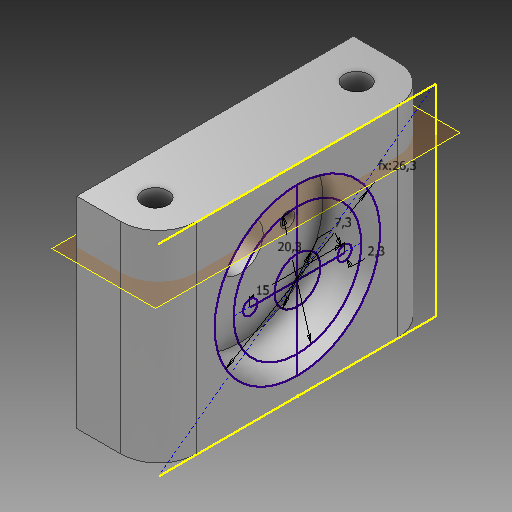
# Autodesk Inventor part: motor_mount_edge
Saved by Autodesk Inventor 2020 (Build 240168000, 168)
## iProperties
Created: 2024-09-09
Part Number: motor_mount_edge
Material: Типовые
Document SubType Name: Modeling
Designer: Ivan
Density: 1 g/cm^3
Appearance: Анодированный — светло-серый
Высота: 32,000 мм
Author: Ivan
Autodesk Inventor part; units mm, degrees
ref_plane "YZ Plane" through (0, 0, 0) normal (1, 0, 0) x (0, 1, 0)
ref_plane "XZ Plane" through (0, 0, 0) normal (0, 1, 0) x (-1, 0, 0)
ref_plane "XY Plane" through (0, 0, 0) normal (0, 0, 1) x (1, 0, 0)
sketch "Эскиз1" plane through (0, 0, 0) normal (0, 1, 0) x (-1, 0, 0)
  line L0 (6.5, 22) -> (-6.5, 22)
  line L1 (-6.5, 22) -> (-6.5, -22)
  line L2 (-6.5, -22) -> (6.5, -22)
  line L3 (6.5, -22) -> (6.5, 22)
  line L4 (-6.5, 22) -> (6.5, -22) construction
  line L5 (0, 22) -> (0, -22) construction
  circle A0 centre (0, 16) radius 2
  line L6 (6.5, 0) -> (-6.5, 0) construction
  circle A1 centre (0, -16) radius 2
  point P0 (0, 0)
  point P1 (0, 0)
  dimension "d0" = 13
  dimension "d1" = 44
  dimension "d2" = 16
  dimension "d3" = 4
  constraints: 14 end point, 5 midpoint, 2 centre point, 2 coincident, 2 parallel, 1 horizontal, 1 perpendicular, 1 point on line, 1 symmetric about line, 1 other
  measures "d0" distance of L2.end L1.end
  measures "d1" distance of L0.end L1.end
  measures "d2" distance of point (0, 0) point (0, 16)
  measures "d3" diameter of A0
extrude "Выдавливание1" add sketch "Эскиз1" along normal blind 32
sketch "Эскиз2" plane through (6.5, 0, 22) normal (1, 0, 0) x (0, 0, -1)
  line L0 (0, 32) -> (44, 32) projected
  line L1 (44, 0) -> (0, 0) projected
  line L2 (44, 32) -> (0, 0) construction
  circle A0 centre (22, 16) radius 10.15
  line L3 (11.85, 16) -> (32.15, 16) construction
  circle A1 centre (14.5, 16) radius 1.15
  circle A2 centre (29.5, 16) radius 1.15
  line L4 (14.5, 16) -> (29.5, 16)
  circle A3 centre (22, 16) radius 13.15
  line L5 (22, 29.15) -> (22, 2.85)
  line L6 (44, 0) -> (44, 32) projected
  circle A4 centre (22, 16) radius 3.65
  point P0 (22, 0)
  dimension "d9" = 20.3
  dimension "d10" = 2.3
  dimension "d11" = 15
  dimension "d17" = 7.3
  dimension "d21" = 26.3
  constraints: 8 end point, 5 centre point, 4 midpoint, 4 point on circle, 2 coincident, 2 point on line, 1 collinear, 1 equal radius, 1 horizontal, 1 parallel
  measures "d9" diameter of A0
  measures "d10" diameter of A2
  measures "d11" distance of L4.start L4.end
  measures "d17" diameter of A4
  measures "d21" diameter of A3
extrude "Выдавливание3" cut sketch "Эскиз2" against normal through all contours A4 L4 L5 | L5 L4 A4 | A4 L4 L5 | L5 L4 A4 | A1 | A2
extrude "Выдавливание4" cut sketch "Эскиз2" against normal blind 9
ref_plane "РабПлоскость1" through (0, 25, 0) normal (0, 1, 0) x (1, 0, 0)
sketch "Эскиз3" plane through (0, 25, 0) normal (0, 1, 0) x (1, 0, 0)
  circle A0 centre (0, -16) radius 2 projected
  circle A1 centre (0, 16) radius 2 projected
  point P0 (0, 0)
extrude "Выдавливание5" add sketch "Эскиз3" against normal blind 16
fillet "Сопряжение1" radius 6 2 edges at (6.5, 16, 22) (6.5, 16, -22)
chamfer "Фаска1" distance 1.2 angle 45 2 edges at (-6.5, 16, -6.35) (-6.5, 16, 8.65)
